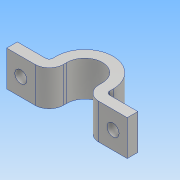
# Autodesk Inventor part: Top_Cable Tie
Saved by Autodesk Inventor 2018.1 (Build 221171000, 171)
## iProperties
Created: 2019-03-23
Part Number: Top_Cable Tie
Material: Aluminum 6061
Document SubType Name: Modeling
Designer: James
Density: 2.7 g/cm^3
Appearance: Aluminum - Flat
Author: James
Autodesk Inventor part; units mm, degrees
ref_plane "YZ Plane" through (0, 0, 0) normal (1, 0, 0) x (0, 1, 0)
ref_plane "XZ Plane" through (0, 0, 0) normal (0, 1, 0) x (-1, 0, 0)
ref_plane "XY Plane" through (0, 0, 0) normal (0, 0, 1) x (1, 0, 0)
sketch "Sketch1" plane through (0, 0, 0) normal (0, 0, 1) x (1, 0, 0)
  line L0 (0, 0) -> (12, 0)
  line L1 (12, 0) -> (12, 3)
  line L2 (12, 3) -> (0, 3)
  line L3 (0, 3) -> (0, 0)
  line L4 (12, 0) -> (9, 0)
  line L5 (9, 0) -> (9, 5)
  line L6 (9, 5) -> (12, 5)
  line L7 (12, 5) -> (12, 0)
  line L8 (22, 5) -> (25, 5)
  line L9 (25, 5) -> (25, 0)
  line L10 (25, 0) -> (22, 0)
  line L11 (22, 0) -> (22, 5)
  line L12 (22, 0) -> (34, 0)
  line L13 (34, 0) -> (34, 3)
  line L14 (34, 3) -> (22, 3)
  line L15 (22, 3) -> (22, 0)
  arc A0 (25, 5) -> (9, 5) centre (17, 5) ccw
  arc A1 (22, 5) -> (12, 5) centre (17, 5) ccw
  dimension "d0" = 3
  dimension "d1" = 3
  dimension "d2" = 12
  dimension "d3" = 12
  dimension "d4" = 5
  dimension "d5" = 5
  constraints: 34 end point, 8 parallel, 4 horizontal, 4 horizontal alignment, 4 perpendicular, 4 point on circle, 3 point on line, 2 centre point, 1 coincident
  measures "d0" distance of L12.end L13.end
  measures "d1" distance between parallel lines of L7 L5
  measures "d2" distance of L0.start L0.end
  measures "d3" distance of L10.end L12.end
  measures "d4" radius of A1
  measures "d5" distance from line of L0 A0.centre
extrude "Extrusion1" add sketch "Sketch1" along normal mid plane 10
fillet "Fillet1" radius 1 2 edges at (25, 3, 0) (9, 3, 0)
fillet "Fillet2" radius 4 2 edges at (22, 0, 0) (12, 0, 0)
sketch "Sketch2" plane through (0, 3, 5) normal (0, 1, 0) x (1, 0, 0)
  line L0 (0, 10) -> (0, 0) projected
  line L1 (0, 10) -> (8, 10) projected
  line L2 (26, 10) -> (34, 10) projected
  point P0 (0, 5)
  point P1 (4, 5)
  point P2 (30, 5)
  point P3 (0, 5)
  point P4 (4, 10)
  point P5 (30, 10)
  dimension "d10" = 26
  constraints: 3 midpoint, 2 horizontal alignment, 2 vertical alignment
  measures "d10" distance of point (30, 5) point (4, 5)
hole "Hole1" at (4, 3, 0) at (30, 3, 0) direction (0, -1, 0) diameter 3.4 end through all clearance for "Flat Head Machine Screw" size "M3" standard "Ansi Metric M Profile"
equation "\"d1\" = d0"
equation "\"d3\" = d2"
body "Solid1"
